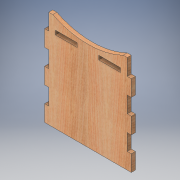
# Autodesk Inventor part: right side
Saved by Autodesk Inventor 2016 (Build 200138000, 138)
## iProperties
Created: 2017-02-03
Part Number: right side
Material: Wood (Birch)
Document SubType Name: Modeling
Designer: jwillauer
Density: 0.55 g/cm^3
Appearance: Birch - Natural Polished
Author: jwillauer
Autodesk Inventor part; units mm, degrees
ref_plane "YZ Plane" through (0, 0, 0) normal (1, 0, 0) x (0, 1, 0)
ref_plane "XZ Plane" through (0, 0, 0) normal (0, 1, 0) x (-1, 0, 0)
ref_plane "XY Plane" through (0, 0, 0) normal (0, 0, 1) x (1, 0, 0)
sketch "Sketch1" plane through (0, 0, 0) normal (0, 0, 1) x (1, 0, 0)
  line L0 (1033.8246, 340.1521) -> (1033.8246, -117.0479)
  line L1 (627.4246, -117.0479) -> (627.4246, 340.1521)
  line L2 (627.4246, -117.0479) -> (1033.8246, -117.0479)
  arc A0 (665.5246, 340.1521) -> (995.7246, 340.1521) centre (830.6246, 678.8187) ccw
  line L3 (627.4246, 340.1521) -> (665.5246, 340.1521)
  line L4 (995.7246, 340.1521) -> (1033.8246, 340.1521)
  point P0 (0, 0)
  dimension "d0" = 406.4
  dimension "d1" = 457.2
  constraints: 10 end point, 3 horizontal, 2 perpendicular, 2 point on circle, 1 centre point, 1 parallel
  measures "d0" distance of L1.end L0.start
  measures "d1" distance of L0.start L0.end
extrude "Extrusion1" add sketch "Sketch1" along normal blind 19.05
sketch "Sketch2" plane through (0, 0, 19.05) normal (0, 0, 1) x (1, 0, 0)
  line L0 (1033.8246, 340.1521) -> (627.4246, 340.1521) projected
  line L1 (627.4246, -117.0479) -> (-960.0754, -117.0479) projected
  line L2 (627.4246, 340.1521) -> (646.4746, 340.1521)
  line L3 (646.4746, 340.1521) -> (646.4746, -117.0479)
  line L4 (646.4746, -117.0479) -> (627.4246, -117.0479)
  line L5 (627.4246, -117.0479) -> (627.4246, 340.1521)
  line L6 (1033.8246, -117.0479) -> (1033.8246, 340.1521) projected
  line L7 (1033.8246, 340.1521) -> (1014.7746, 340.1521)
  line L8 (1014.7746, 340.1521) -> (1014.7746, -117.0479)
  line L9 (1014.7746, -117.0479) -> (1033.8246, -117.0479)
  line L10 (1033.8246, -117.0479) -> (1033.8246, 340.1521)
  line L11 (627.4246, 340.1521) -> (627.4246, -117.0479) projected
  line L12 (627.4246, 263.9521) -> (646.4746, 263.9521)
  line L13 (1014.7746, 263.9521) -> (1033.8246, 263.9521)
  line L14 (627.4246, 187.7521) -> (646.4746, 187.7521)
  line L15 (1014.7746, 187.7521) -> (1033.8246, 187.7521)
  line L16 (627.4246, 111.5521) -> (646.4746, 111.5521)
  line L17 (1014.7746, 111.5521) -> (1033.8246, 111.5521)
  line L18 (627.4246, 35.3521) -> (646.4746, 35.3521)
  line L19 (1014.7746, 35.3521) -> (1033.8246, 35.3521)
  line L20 (1033.8246, -40.8479) -> (1014.7746, -40.8479)
  line L21 (646.4746, -40.8479) -> (627.4246, -40.8479)
  point P0 (0, 0)
  dimension "d7" = 19.05
  dimension "d8" = 19.05
  constraints: 36 end point, 18 point on line, 12 perpendicular, 4 midpoint, 4 parallel, 2 horizontal
  measures "d7" distance between parallel lines of L3 L5
  measures "d8" distance between parallel lines of L6 L8
extrude "Extrusion2" cut sketch "Sketch2" against normal blind 19.05 contours L6 L13 L8 L0 | L3 L12 L5 L0 | L6 L17 L8 L15 | L3 L16 L5 L14 | L6 L20 L8 L19 | L3 L21 L5 L18
sketch "Sketch3" plane through (0, 0, 19.05) normal (0, 0, 1) x (1, 0, 0)
  line L0 (1131.5205, 302.0521) -> (511.2286, 302.0521)
  line L1 (1014.7746, 340.1521) -> (995.7246, 340.1521) projected
  line L2 (1127.4261, 283.0021) -> (305.147, 283.0021)
  line L3 (830.6246, 74.0239) -> (830.6246, 388.6053)
  line L4 (1033.8246, 187.7521) -> (1033.8246, 263.9521) projected
  line L5 (983.0246, 283.0021) -> (881.4246, 283.0021)
  line L6 (881.4246, 283.0021) -> (881.4246, 263.9521)
  line L7 (881.4246, 263.9521) -> (983.0246, 263.9521)
  line L8 (983.0246, 263.9521) -> (983.0246, 283.0021)
  line L9 (1014.7746, 263.9521) -> (1014.7746, 340.1521) projected
  line L10 (678.2246, 283.0021) -> (779.8246, 283.0021)
  line L11 (779.8246, 283.0021) -> (779.8246, 263.9521)
  line L12 (779.8246, 263.9521) -> (678.2246, 263.9521)
  line L13 (678.2246, 263.9521) -> (678.2246, 283.0021)
  line L14 (646.4746, 340.1521) -> (646.4746, 263.9521) projected
  point P0 (0, 0)
  dimension "d24" = 38.1
  dimension "d25" = 19.05
  dimension "d26" = 203.2
  dimension "d27" = 31.75
  dimension "d28" = 101.6
  dimension "d29" = 19.05
  dimension "d30" = 31.75
  dimension "d31" = 101.6
  dimension "d32" = 19.05
  constraints: 22 end point, 4 horizontal, 4 parallel, 2 perpendicular, 2 point on line, 1 vertical
  measures "d24" distance between parallel lines of L0 L1
  measures "d25" distance between parallel lines of L2 L0
  measures "d26" distance between parallel lines of L3 L4
  measures "d27" distance between parallel lines of L8 L9
  measures "d28" distance of L6.end L7.end
  measures "d29" distance between parallel lines of L2 L7
  measures "d30" distance between parallel lines of L13 L14
  measures "d31" distance of L11.end L12.end
  measures "d32" distance between parallel lines of L10 L12
extrude "Extrusion3" cut sketch "Sketch3" against normal blind 25.4 contours L8 L7 L6 L2 | L11 L12 L13 L2
body "Solid1"
